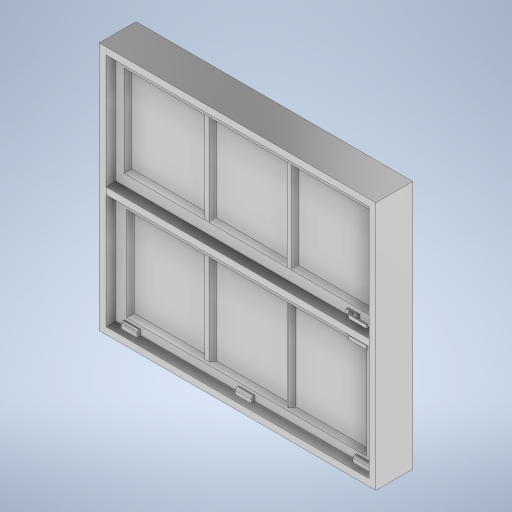
# Autodesk Inventor part: Window
Saved by Autodesk Inventor 2023 (Build 270158000, 158)
## iProperties
Created: 2022-10-13
Part Number: Window
Material: Nickel-Copper Alloy 400
Document SubType Name: Modeling
Designer: mliu-23
Density: 8.83 g/cm^3
Appearance: Chrome - Polished
Author: mliu-23
Autodesk Inventor part; units mm, degrees
ref_plane "YZ Plane" through (0, 0, 0) normal (1, 0, 0) x (0, 1, 0)
ref_plane "XZ Plane" through (0, 0, 0) normal (0, 1, 0) x (-1, 0, 0)
sketch "Sketch1" plane through (0, 0, 0) normal (0, 0, 1) x (1, 0, 0)
  line L0 (-762, -685.8) -> (762, -685.8)
  line L1 (762, -685.8) -> (762, 685.8)
  line L2 (762, 685.8) -> (-762, 685.8)
  line L3 (-762, 685.8) -> (-762, -685.8)
  line L4 (-762, -685.8) -> (762, 685.8) construction
  line L5 (762, -685.8) -> (-762, 685.8) construction
  point P0 (0, 0)
  dimension "d0" = 1524
  dimension "d1" = 1371.6
  constraints: 12 end point, 2 midpoint, 2 parallel, 1 horizontal, 1 perpendicular
  measures "d0" distance of L2.end L1.end
  measures "d1" distance of L1.end L0.end
extrude "Extrusion1" add sketch "Sketch1" along normal mid plane 203.2
sketch "Sketch2" plane through (0, 0, 101.6) normal (0, 0, 1) x (1, 0, 0)
  line L0 (723.9, -647.7) -> (-723.9, -647.7)
  line L1 (-723.9, -647.7) -> (-723.9, 647.7)
  line L2 (-723.9, 647.7) -> (723.9, 647.7)
  line L3 (723.9, 647.7) -> (723.9, -647.7)
  line L4 (723.9, -647.7) -> (-723.9, 647.7) construction
  line L5 (-723.9, -647.7) -> (723.9, 647.7) construction
  line L6 (762, 685.8) -> (-762, 685.8) projected
  line L7 (-762, 685.8) -> (-762, -685.8) projected
  point P0 (0, 0)
  dimension "d4" = 38.1
  dimension "d5" = 38.1
  constraints: 12 end point, 2 midpoint, 2 parallel, 1 horizontal, 1 perpendicular
  measures "d4" distance between parallel lines of L6 L2
  measures "d5" distance between parallel lines of L7 L1
extrude "Extrusion2" cut sketch "Sketch2" against normal blind 50.8
sketch "Sketch4" plane through (0, 0, 50.8) normal (0, 0, 1) x (1, 0, 0)
  line L0 (723.9, -19.05) -> (-723.9, -19.05)
  line L1 (-723.9, -19.05) -> (-723.9, 19.05)
  line L2 (-723.9, 19.05) -> (723.9, 19.05)
  line L3 (723.9, 19.05) -> (723.9, -19.05)
  line L4 (723.9, -19.05) -> (-723.9, 19.05) construction
  line L5 (-723.9, -19.05) -> (723.9, 19.05) construction
  line L6 (-723.9, -647.7) -> (-723.9, 647.7) projected
  point P0 (0, 0)
  point P1 (-723.9, 0)
  dimension "d8" = 38.1
  constraints: 12 end point, 4 midpoint, 2 parallel, 1 horizontal, 1 perpendicular
  measures "d8" distance of L0.end L1.end
extrude "Extrusion3" add sketch "Sketch4" along normal blind 50.8 separate body
sketch "Sketch5" plane through (0, 0, 50.8) normal (0, 0, 1) x (1, 0, 0)
  line L0 (-723.9, 647.7) -> (723.9, 647.7) projected
  line L1 (-723.9, -647.7) -> (-723.9, 647.7) projected
  line L2 (723.9, -647.7) -> (-723.9, -647.7) projected
  line L3 (723.9, 647.7) -> (723.9, -647.7) projected
  line L4 (-723.9, -19.05) -> (723.9, -19.05) projected
  line L5 (723.9, 19.05) -> (-723.9, 19.05) projected
  line L6 (660.4, -584.2) -> (-660.4, -584.2)
  line L7 (-660.4, -584.2) -> (-660.4, -82.55)
  line L8 (-660.4, -82.55) -> (660.4, -82.55)
  line L9 (660.4, -82.55) -> (660.4, -584.2)
  line L10 (660.4, -584.2) -> (-660.4, -82.55) construction
  line L11 (-660.4, -584.2) -> (660.4, -82.55) construction
  line L12 (-762, 685.8) -> (-762, -685.8) construction
  line L13 (-762, 0) -> (762, 0) construction
  line L14 (762, -685.8) -> (762, 685.8) construction
  line L15 (660.4, 584.2) -> (-660.4, 584.2)
  line L16 (-660.4, 584.2) -> (-660.4, 82.55)
  line L17 (-660.4, 82.55) -> (660.4, 82.55)
  line L18 (660.4, 82.55) -> (660.4, 584.2)
  point P0 (0, 0)
  point P1 (0, -333.375)
  point P2 (0, -19.05)
  dimension "d11" = 63.5
  dimension "d12" = 63.5
  dimension "d13" = 63.5
  constraints: 22 end point, 5 midpoint, 4 symmetric about line, 2 parallel, 1 horizontal, 1 perpendicular, 1 vertical alignment
  measures "d11" distance between parallel lines of L1 L7
  measures "d12" distance between parallel lines of L2 L6
  measures "d13" distance between parallel lines of L4 L8
extrude "Extrusion4" cut sketch "Sketch5" against normal blind 25.4 contours L6 L7 L8 L9 | L18 L17 L16 L15 bodies 1
sketch "Sketch6" plane through (0, 0, 25.4) normal (0, 0, 1) x (1, 0, 0)
  line L0 (660.4, -584.2) -> (-660.4, -584.2) projected
  line L1 (-660.4, -82.55) -> (660.4, -82.55) projected
  line L2 (-245.5333, -584.2) -> (-207.4333, -584.2)
  line L3 (-207.4333, -584.2) -> (-207.4333, -82.55)
  line L4 (-207.4333, -82.55) -> (-245.5333, -82.55)
  line L5 (-245.5333, -82.55) -> (-245.5333, -584.2)
  line L6 (207.4333, -584.2) -> (245.5333, -584.2)
  line L7 (245.5333, -584.2) -> (245.5333, -82.55)
  line L8 (245.5333, -82.55) -> (207.4333, -82.55)
  line L9 (207.4333, -82.55) -> (207.4333, -584.2)
  line L10 (660.4, 82.55) -> (-660.4, 82.55) projected
  line L11 (-660.4, 584.2) -> (660.4, 584.2) projected
  line L12 (207.4333, 82.55) -> (245.5333, 82.55)
  line L13 (245.5333, 82.55) -> (245.5333, 584.2)
  line L14 (245.5333, 584.2) -> (207.4333, 584.2)
  line L15 (207.4333, 584.2) -> (207.4333, 82.55)
  line L16 (-245.5333, 82.55) -> (-207.4333, 82.55)
  line L17 (-207.4333, 82.55) -> (-207.4333, 584.2)
  line L18 (-207.4333, 584.2) -> (-245.5333, 584.2)
  line L19 (-245.5333, 584.2) -> (-245.5333, 82.55)
  line L20 (660.4, -584.2) -> (-660.4, -584.2) projected
  line L21 (-660.4, -333.375) -> (-245.5333, -333.375) construction
  line L22 (-207.4333, -333.375) -> (207.4333, -333.375) construction
  line L23 (245.5333, -333.375) -> (660.4, -333.375) construction
  line L24 (660.4, -82.55) -> (660.4, -584.2) construction
  line L25 (-660.4, -584.2) -> (-660.4, -82.55) construction
  point P0 (0, 0)
  dimension "d16" = 38.1
  dimension "d17" = 38.1
  constraints: 38 end point, 12 point on line, 8 parallel, 6 midpoint, 5 horizontal, 4 coincident, 4 perpendicular, 2 collinear
  measures "d16" distance between parallel lines of L3 L5
  measures "d17" distance between parallel lines of L7 L9
extrude "Extrusion5" add sketch "Sketch6" along normal blind 25.4 separate body contours L0 L9 L1 L7 | L0 L5 L1 L3 | L10 L15 L11 L13 | L10 L19 L11 L17
draft "FaceDraft1" angle 30 pull direction (0, 0, 1) faces at (-220.1333, -584.2, 33.8667) (-660.4, -249.7667, 42.3333) (220.1333, -82.55, 33.8667) (660.4, -416.9833, 42.3333) (660.4, 249.7667, 42.3333) (-220.1333, 82.55, 33.8667) (220.1333, 584.2, 33.8667) (-660.4, 416.9833, 42.3333) fixed edges at (0, -584.2, 25.4) (-660.4, -333.375, 50.8) (0, -82.55, 50.8) (660.4, -333.375, 50.8) (660.4, 333.375, 25.4) (0, 82.55, 50.8) (0, 584.2, 50.8) (-660.4, 333.375, 25.4) (226.4833, -584.2, 25.4) (-226.4833, -584.2, 25.4) (226.4833, -82.55, 50.8) (-226.4833, -82.55, 50.8) (226.4833, 82.55, 50.8) (-226.4833, 82.55, 50.8) (226.4833, 584.2, 50.8) (-226.4833, 584.2, 50.8)
draft "FaceDraft2" angle 30 pull direction (0, 0, 1) faces at (-207.4333, -416.9833, 33.8667) (-245.5333, -249.7667, 33.8667) (-245.5333, 416.9833, 33.8667) (-207.4333, 249.7667, 33.8667) (207.4333, 416.9833, 33.8667) (245.5333, 249.7667, 33.8667) (207.4333, -249.7667, 33.8667) (245.5333, -416.9833, 33.8667) fixed edges at (-207.4333, -333.375, 50.8) (-245.5333, -333.375, 25.4) (-245.5333, 333.375, 25.4) (-207.4333, 333.375, 50.8) (207.4333, 333.375, 25.4) (245.5333, 333.375, 50.8) (207.4333, -333.375, 25.4) (245.5333, -333.375, 25.4)
sketch "Sketch7" plane through (0, 0, 50.8) normal (0, 0, 1) x (1, 0, 0)
  line L0 (-675.0647, 584.2) -> (675.0647, 584.2) projected
  line L1 (675.0647, 584.2) -> (675.0647, 82.55) projected
  line L2 (675.0647, 82.55) -> (-675.0647, 82.55) projected
  line L3 (-675.0647, 82.55) -> (-675.0647, 584.2) projected
  line L4 (-660.4, -598.8647) -> (-660.4, -82.55) projected
  line L5 (-660.4, -82.55) -> (660.4, -82.55) projected
  line L6 (660.4, -82.55) -> (660.4, -598.8647) projected
  line L7 (660.4, -598.8647) -> (-660.4, -598.8647) projected
  line L8 (-723.9, 647.7) -> (723.9, 647.7) projected
  line L9 (-723.9, -647.7) -> (-723.9, 647.7) projected
  line L10 (723.9, -647.7) -> (-723.9, -647.7) projected
  line L11 (723.9, 647.7) -> (723.9, -647.7) projected
  line L12 (-721.36, 645.16) -> (721.36, 645.16)
  line L13 (721.36, 645.16) -> (721.36, -645.16)
  line L14 (721.36, -645.16) -> (-721.36, -645.16)
  line L15 (-721.36, -645.16) -> (-721.36, 645.16)
  line L16 (-723.9, -19.05) -> (723.9, -19.05) projected
  line L17 (723.9, 19.05) -> (-723.9, 19.05) projected
  line L18 (-723.9, -21.59) -> (723.9, -21.59)
  line L19 (723.9, 21.59) -> (-723.9, 21.59)
  point P0 (0, 0)
  point P1 (-721.36, 21.59)
  point P2 (721.36, 21.59)
  point P3 (-721.36, 19.05)
  point P4 (721.36, 19.05)
  point P5 (721.36, -21.59)
  point P6 (-721.36, -21.59)
  point P7 (721.36, -19.05)
  point P8 (-721.36, -19.05)
  dimension "d22" = 2.54
  dimension "d23" = 2.54
  dimension "d24" = 2.54
  constraints: 12 end point, 2 parallel, 3 other
  measures "d22" distance between parallel lines of L9 L15
  measures "d23" distance between parallel lines of L16 L18
  measures "d24" distance between parallel lines of L17 L19
extrude "Extrusion6" cut sketch "Sketch7" against normal blind 25.4 contours L8 L11 L19 L13 L12 L15 L9 | L19 L13 L17 L15 | L18 L15 L14 L13 L11 L10 L9 | L16 L13 L18 L15 bodies 1
sketch "Sketch8" plane through (0, 0, 50.8) normal (0, 0, 1) x (1, 0, 0)
  line L0 (723.9, -647.7) -> (-723.9, -647.7) projected
  line L1 (-723.9, -647.7) -> (-723.9, 647.7) projected
  line L2 (-673.1, -647.7) -> (-584.2, -647.7)
  line L3 (-584.2, -647.7) -> (-584.2, -615.95)
  line L4 (-584.2, -615.95) -> (-673.1, -615.95)
  line L5 (-673.1, -615.95) -> (-673.1, -647.7)
  line L6 (603.25, -647.7) -> (692.15, -647.7)
  line L7 (692.15, -647.7) -> (692.15, -615.95)
  line L8 (692.15, -615.95) -> (603.25, -615.95)
  line L9 (603.25, -615.95) -> (603.25, -647.7)
  line L10 (-44.45, -647.7) -> (44.45, -647.7)
  line L11 (44.45, -647.7) -> (44.45, -615.95)
  line L12 (44.45, -615.95) -> (-44.45, -615.95)
  line L13 (-44.45, -615.95) -> (-44.45, -647.7)
  line L14 (723.9, 647.7) -> (723.9, -647.7) projected
  line L15 (-723.9, -19.05) -> (723.9, -19.05) construction
  line L16 (-723.9, 0) -> (723.9, 0) construction
  line L17 (723.9, -19.05) -> (723.9, 19.05) construction
  line L18 (-673.1, 647.7) -> (-584.2, 647.7)
  line L19 (-584.2, 647.7) -> (-584.2, 615.95)
  line L20 (-584.2, 615.95) -> (-673.1, 615.95)
  line L21 (-673.1, 615.95) -> (-673.1, 647.7)
  line L22 (692.15, 647.7) -> (692.15, 615.95)
  line L23 (692.15, 615.95) -> (603.25, 615.95)
  line L24 (603.25, 615.95) -> (603.25, 647.7)
  line L25 (44.45, 647.7) -> (44.45, 615.95)
  line L26 (44.45, 615.95) -> (-44.45, 615.95)
  line L27 (-44.45, 615.95) -> (-44.45, 647.7)
  line L28 (721.36, 645.16) -> (-721.36, 645.16) construction
  line L29 (-673.1, 647.7) -> (-584.2, 647.7)
  line L30 (-44.45, 647.7) -> (44.45, 647.7)
  line L31 (-723.9, 647.7) -> (723.9, 647.7) projected
  line L32 (603.25, 647.7) -> (692.15, 647.7)
  point P0 (0, 0)
  point P1 (-673.1, -631.825)
  point P2 (-673.1, 631.825)
  dimension "d27" = 50.8
  dimension "d28" = 88.9
  dimension "d29" = 31.75
  dimension "d30" = 31.75
  dimension "d31" = 539.75
  constraints: 52 end point, 13 symmetric about line, 8 parallel, 7 point on line, 3 collinear, 3 horizontal, 3 midpoint, 3 perpendicular
  measures "d27" distance from line of point (-673.1, -631.825) L1
  measures "d28" distance of L3.end L4.end
  measures "d29" distance of L4.end L2.start
  measures "d30" distance between parallel lines of L14 L7
  measures "d31" distance between parallel lines of L13 L3
extrude "Extrusion7" add sketch "Sketch8" along normal blind 19.05 separate body contours L0 L9 L8 L7 | L22 L23 L24 L31 | L0 L13 L12 L11 | L25 L26 L27 L30 | L0 L5 L4 L3 | L19 L20 L21 L18
fillet "Fillet1" radius 12.7 6 edges at (-628.65, -615.95, 69.85) (0, -615.95, 69.85) (647.7, -615.95, 69.85) (647.7, 615.95, 69.85) (0, 615.95, 69.85) (-628.65, 615.95, 69.85)
sketch "Sketch9" plane through (0, 0, 50.8) normal (0, 0, 1) x (1, 0, 0)
  line L0 (558.8, -40.0647) -> (622.3, -40.0647)
  line L1 (622.3, -40.0647) -> (622.3, -59.1147)
  line L2 (622.3, -59.1147) -> (558.8, -59.1147)
  line L3 (558.8, -59.1147) -> (558.8, -40.0647)
  line L4 (723.9, 647.7) -> (723.9, -647.7) projected
  line L5 (-645.7353, -97.2147) -> (645.7353, -97.2147) projected
  line L6 (762, -685.8) -> (762, 685.8) construction
  line L7 (762, 0) -> (-762, 0) construction
  line L8 (-762, 685.8) -> (-762, -685.8) construction
  line L9 (558.8, 40.0647) -> (622.3, 40.0647)
  line L10 (622.3, 40.0647) -> (622.3, 59.1147)
  line L11 (622.3, 59.1147) -> (558.8, 59.1147)
  line L12 (558.8, 59.1147) -> (558.8, 40.0647)
  point P0 (0, 0)
  point P1 (622.3, -49.5897)
  point P2 (558.8, -49.5897)
  dimension "d35" = 63.5
  dimension "d36" = 101.6
  dimension "d37" = 19.05
  dimension "d38" = 38.1
  constraints: 18 end point, 4 midpoint, 4 symmetric about line, 2 parallel, 1 horizontal, 1 perpendicular
  measures "d35" distance of point (622.3, -49.59) point (558.8, -49.59)
  measures "d36" distance between parallel lines of L4 L1
  measures "d37" distance of L2.end L0.start
  measures "d38" distance between parallel lines of L5 L2
extrude "Extrusion8" add sketch "Sketch9" along normal blind 12.7 separate body
sketch "Sketch10" plane through (0, 0, 63.5) normal (0, 0, 1) x (1, 0, 0)
  point P0 (0, 0)
sketch "Sketch11" plane through (558.8, -59.1147, 50.8) normal (0, -1, 0) x (1, 0, 0)
  line L0 (165.1, -25.4) -> (-1282.7, -25.4) projected
  line L1 (63.5, 12.7) -> (0, 12.7) projected
  line L2 (63.5, 0) -> (0, 0) projected
  line L3 (0, 0) -> (0, 12.7) projected
  line L4 (63.5, 12.7) -> (0, 12.7) projected
  line L5 (63.5, 0) -> (63.5, 12.7) projected
  line L6 (63.5, 12.7) -> (0, 12.7) projected
  arc A0 (34.7447, 31.9938) -> (21.0841, 12.7) centre (41.6152, 12.6464) ccw
  line L7 (35.8072, 32.1768) -> (133.4816, 32.1768)
  arc A1 (43.7111, 20.8584) -> (37.1866, 12.7) centre (45.9464, 12.3826) ccw
  line L8 (133.4816, 25.9019) -> (133.4816, 32.1768)
  arc A2 (35.8072, 32.1768) -> (34.7447, 31.9938) centre (35.8072, 29.0018) ccw
  line L9 (43.7111, 20.8584) -> (133.4816, 25.9019)
  point P0 (-558.8, -50.8)
  point P1 (35.2837, 32.1768)
  point P2 (37.1866, 12.7)
  dimension "d42" = 3.175
  constraints: 7 point on circle, 6 end point, 3 centre point, 3 point on line, 2 tangent, 1 horizontal
  measures "d42" radius of A2
extrude "Extrusion9" add sketch "Sketch11" against normal blind 19.05 separate body contours L1 A0 A2 L7 L8 L9 A1
ref_plane "Work Plane1" through (-723.9, 0, 50.8) normal (0, -1, 0) x (1, 0, 0)
mirror "Mirror1" about plane through (-723.9, 0, 50.8) normal (0, -1, 0) of "Extrusion9" bodies 6
body "Solid1"
body "Solid2"
body "Solid3"
body "Solid4"
body "Solid5"
body "Solid6"
